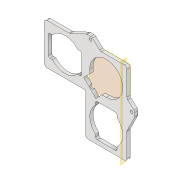
# Autodesk Inventor part: 20_Cube_Insert_Openflexure_Adapter
Saved by Autodesk Inventor 2019 (Build 230136000, 136)
## iProperties
Created: 2019-08-12
Part Number: 20_Cube_Insert_Openflexure_Adapter
Material: Generic
Document SubType Name: Modeling
Designer: diederichbenedict
Density: 1 g/cm^3
Appearance: White
Author: diederichbenedict
Autodesk Inventor part; units mm, degrees
ref_plane "YZ Plane" through (0, 0, 0) normal (1, 0, 0) x (0, 1, 0)
ref_plane "XZ Plane" through (0, 0, 0) normal (0, 1, 0) x (-1, 0, 0)
ref_plane "XY Plane" through (0, 0, 0) normal (0, 0, 1) x (1, 0, 0)
ref_plane "Work Plane1" through (0, 0, 0) normal (0, 0, 1) x (1, 0, 0)
sketch "Sketch1" plane through (0, 0, 0) normal (0, 0, 1) x (1, 0, 0)
  line L0 (-16.9, -16.9) -> (-16.9, 16.9) construction
  line L1 (-16.9, 16.9) -> (16.9, 16.9) construction
  line L2 (16.9, 16.9) -> (16.9, -16.9) construction
  line L3 (16.9, -16.9) -> (-16.9, -16.9) construction
  circle A0 centre (-19.9, 19.9) radius 2.75 construction
  circle A1 centre (19.9, -19.9) radius 2.75 construction
  circle A2 centre (19.9, 19.9) radius 2.75 construction
  circle A3 centre (-19.9, -19.9) radius 2.75 construction
  line L4 (-22.9, 22.9) -> (22.9, 22.9) construction
  line L5 (-22.9, -22.9) -> (-22.9, 22.9) construction
  line L6 (22.9, -22.9) -> (-22.9, -22.9) construction
  line L7 (22.9, 22.9) -> (22.9, -22.9) construction
  circle A4 centre (0, 0) radius 19.9847 construction
  circle A5 centre (30.6716, -19.9141) radius 1.6508 construction
  circle A6 centre (-19.2474, 31.0959) radius 1.649 construction
  line L8 (-11.1833, 28.6006) -> (11.7978, 28.3526) construction
  line L9 (-17.6359, 34.6452) -> (-11.1833, 28.6006) construction
  line L10 (-23.6485, 34.6452) -> (-17.6359, 34.6452) construction
  line L11 (-22.8713, 22.6559) -> (-23.6485, 34.6452) construction
  line L12 (-23.6485, -13.3567) -> (-22.8713, 22.6559) construction
  line L13 (-23.6485, -23.3548) -> (-23.6485, -13.3567) construction
  line L14 (34.3515, -23.3548) -> (-23.6485, -23.3548) construction
  line L15 (34.3515, -17.3548) -> (34.3515, -23.3548) construction
  line L16 (28.3526, -11.7978) -> (34.3515, -17.3548) construction
  line L17 (28.6006, 11.1833) -> (28.3526, -11.7978) construction
  arc A7 (28.6006, 11.1833) -> (11.7978, 28.3526) centre (10.7217, 10.4928) ccw construction
  arc A8 (-24.9, -22.9) -> (-22.9, -24.9) centre (-22.9, -22.9) ccw construction
  arc A9 (-22.9, 24.9) -> (-24.9, 22.9) centre (-22.9, 22.9) ccw construction
  arc A10 (24.9, 22.9) -> (22.9, 24.9) centre (22.9, 22.9) ccw construction
  arc A11 (22.9, -24.9) -> (24.9, -22.9) centre (22.9, -22.9) ccw construction
  line L18 (24.9, 24.9) -> (-74.9, 24.9) construction
  line L19 (-74.9, 24.9) -> (-74.9, -24.9) construction
  line L20 (-74.9, -24.9) -> (24.9, -24.9) construction
  line L21 (24.9, -24.9) -> (24.9, 24.9) construction
  line L22 (24.9, -24.9) -> (-25, -24.9) construction
  line L23 (-25, -24.9) -> (-25, -74.9) construction
  line L24 (-25, -74.9) -> (24.9, -74.9) construction
  line L25 (24.9, -74.9) -> (24.9, -24.9) construction
  line L26 (-74.9, 24.9) -> (-25, 24.9)
  line L27 (-25, 24.9) -> (-25, -24.9)
  line L28 (-25, -24.9) -> (-74.9, -24.9)
  line L29 (-74.9, -24.9) -> (-74.9, 24.9)
  line L30 (-25, -74.9) -> (24.9, -74.9)
  line L31 (24.9, -74.9) -> (24.9, -24.9)
  line L32 (24.9, -24.9) -> (-25, -24.9)
  line L33 (-25, -24.9) -> (-25, -74.9)
  circle A12 centre (0, 0) radius 20
  circle A13 centre (-50, 0) radius 20
  circle A14 centre (0, -50) radius 20
  line L34 (-25, -24.9) -> (24.9, -24.9)
  line L35 (24.9, -24.9) -> (24.9, 24.9)
  line L36 (24.9, 24.9) -> (-25, 24.9)
  line L37 (-25, 24.9) -> (-25, -24.9)
  line L38 (34.3515, -23.3548) -> (12.5761, -67.8407) construction
  line L39 (-24.6505, -24.1243) -> (34.3515, -23.3548) construction
  line L40 (-23.6485, 34.6452) -> (-24.6505, -24.1243) construction
  line L41 (-67.591, 14.0198) -> (-23.6485, 34.6452) construction
  arc A15 (-67.591, 14.0198) -> (-72.2252, 6.8961) centre (-64.1657, 6.7223) ccw construction
  line L42 (-72.3572, -5.3362) -> (-72.2252, 6.8961) construction
  arc A16 (-72.3572, -5.3362) -> (-70.7942, -10.6047) centre (-52.5572, -2.3284) ccw construction
  line L43 (-59.2435, -49.54) -> (-70.7942, -10.6047) construction
  line L44 (-50.8067, -58.1609) -> (-59.2435, -49.54) construction
  arc A17 (-50.8067, -58.1609) -> (-47.0776, -60.4156) centre (-44.5702, -52.0575) ccw construction
  line L45 (-6.8108, -72.2261) -> (-47.0776, -60.4156) construction
  arc A18 (-6.8108, -72.2261) -> (12.5761, -67.8407) centre (0.6863, -60.3238) ccw construction
  circle A19 centre (0, 0) radius 19.9847 construction
  circle A20 centre (-19.2474, 31.0959) radius 1.649 construction
  circle A21 centre (30.6716, -19.9141) radius 1.6508 construction
  line L46 (-11.1833, 28.6006) -> (11.7978, 28.3526) construction
  line L47 (-17.6359, 34.6452) -> (-11.1833, 28.6006) construction
  line L48 (-23.6485, 34.6452) -> (-17.6359, 34.6452) construction
  line L49 (-22.8713, 22.6559) -> (-23.6485, 34.6452) construction
  line L50 (-23.6485, -13.3567) -> (-22.8713, 22.6559) construction
  line L51 (-23.6485, -23.3548) -> (-23.6485, -13.3567) construction
  line L52 (34.3515, -23.3548) -> (-23.6485, -23.3548) construction
  line L53 (34.3515, -17.3548) -> (34.3515, -23.3548) construction
  line L54 (28.3526, -11.7978) -> (34.3515, -17.3548) construction
  line L55 (28.6006, 11.1833) -> (28.3526, -11.7978) construction
  arc A22 (28.6006, 11.1833) -> (11.7978, 28.3526) centre (10.7217, 10.4928) ccw construction
  line L56 (24.9, -42.6637) -> (34.3515, -23.3548)
  line L57 (34.3515, -23.3548) -> (34.3515, -17.3548)
  line L58 (34.3515, -17.3548) -> (24.9, -8.5995)
  line L59 (-17.6359, 34.6452) -> (-7.2331, 24.9)
  line L60 (-17.6359, 34.6452) -> (-23.6485, 34.6452)
  line L61 (-44.4107, 24.9) -> (-23.6485, 34.6452)
  circle A23 centre (-19.2474, 31.0959) radius 1.75
  circle A24 centre (30.6716, -19.9141) radius 1.75
  line L62 (-7.2331, 24.9) -> (-44.4107, 24.9)
  line L63 (-68, 13) -> (-32, 13)
  line L64 (-30, 11) -> (-30, -11)
  line L65 (-32, -13) -> (-68, -13)
  line L66 (-70, -11) -> (-70, 11)
  arc A25 (-68, 13) -> (-70, 11) centre (-68, 11) ccw
  arc A26 (-30, 11) -> (-32, 13) centre (-32, 11) ccw
  arc A27 (-32, -13) -> (-30, -11) centre (-32, -11) ccw
  arc A28 (-70, -11) -> (-68, -13) centre (-68, -11) ccw
  line L67 (24.9, 24.9) -> (-25, -25) construction
  line L68 (24.9, 24.9) -> (95.4693, 24.9) construction
  circle A29 centre (0, -50) radius 20
  arc A30 (6.8961, -72.2252) -> (14.0198, -67.591) centre (6.7223, -64.1657) ccw construction
  line L69 (-5.3362, -72.3572) -> (6.8961, -72.2252) construction
  arc A31 (-10.6047, -70.7942) -> (-5.3362, -72.3572) centre (-2.3284, -52.5572) ccw construction
  line L70 (13, -68) -> (13, -32)
  line L71 (11, -30) -> (-11, -30)
  line L72 (-13, -32) -> (-13, -68)
  line L73 (-11, -70) -> (11, -70)
  arc A32 (11, -70) -> (13, -68) centre (11, -68) ccw
  arc A33 (13, -32) -> (11, -30) centre (11, -32) ccw
  arc A34 (-11, -30) -> (-13, -32) centre (-11, -32) ccw
  arc A35 (-13, -68) -> (-11, -70) centre (-11, -68) ccw
  point P0 (0, 0)
  point P1 (-30, -13)
  point P2 (-30, 13)
  point P3 (-70, -13)
  point P4 (-13, -30)
  point P5 (13, -30)
  point P6 (-13, -70)
  dimension "d0" = 99.8
  dimension "d1" = 50
  dimension "d2" = 40
  dimension "d3" = 40
  dimension "d4" = 50
  dimension "d5" = 40
  dimension "d6" = 50
  dimension "d25" = 3.5
  dimension "d26" = 3.5
  dimension "d28" = 40
  dimension "d29" = 26
  dimension "d30" = 30
  dimension "d32" = 13
  dimension "d33" = 2
  dimension "d34" = 135
  constraints: 76 end point, 22 symmetric about line, 20 point on circle, 19 point on line, 16 centre point, 12 parallel, 8 tangent, 7 horizontal, 7 perpendicular, 3 coincident, 3 collinear, 3 equal radius, 1 equal length, 7 other
  measures "d0" distance of L20.end L19.end
  measures "d1" distance of L23.end L22.end
  measures "d2" diameter of A12
  measures "d3" diameter of A13
  measures "d4" distance of point (0, 0) A13.centre
  measures "d5" diameter of A14
  measures "d6" distance of A14.centre point (0, 0)
  measures "d25" diameter of A23
  measures "d26" diameter of A24
  measures "d28" distance of point (-30, -13) point (-70, -13)
  measures "d29" distance of point (-30, 13) point (-30, -13)
  measures "d30" distance from line of L64 A19.centre
  measures "d32" distance from line of L63 A19.centre
  measures "d33" radius of A25
  measures "d34" angle of L67 L68
extrude "Extrusion1" add sketch "Sketch1" along normal blind 4
ref_plane "Work Plane2" through (20, -74.9, 0) normal (1, 0, 0) x (0, 0, -1)
sketch "Sketch2" plane through (20, -74.9, 0) normal (1, 0, 0) x (0, 0, -1)
  line L0 (2.5, 97.55) -> (0, 97.55)
  line L1 (2.5, 92.05) -> (0, 92.05)
  line L2 (0, 94.9) -> (-4, 94.9) projected
  circle A0 centre (-1, 94.9) radius 2.45
  line L3 (1.45, 94.9) -> (-3.45, 94.9)
  line L4 (0, 0) -> (0, 99.8) construction
  point P0 (0, 74.9)
  dimension "d10" = 4.9
  dimension "d11" = 1
  constraints: 6 end point, 2 horizontal, 2 point on circle, 2 point on line, 1 centre point, 4 other
  measures "d10" diameter of A0
  measures "d11" distance from line of L4 A0.centre
revolve "Revolution1" cut sketch "Sketch2" angle 360 about axis through (20, 20, -1.45) along (0, 0, 1) picked at (-2.2763, 95.0954) contours L2 A0 L3
pattern_linear "Rectangular Pattern1" count 2 spacing 40 along (0, -1, 0) count 2 spacing 40 along (-1, 0, 0) of "Revolution1"
pattern_linear "Rectangular Pattern2" count 2 spacing 50 along (0, -1, 0) count 2 spacing 50 along (-1, 0, 0) of "Revolution1", "Rectangular Pattern1"
fillet "Fillet1" radius 3 14 edges at (-25, -24.9, 2) (-25, -74.9, 2) (24.9, -74.9, 2) (24.9, -42.6637, 2) (34.3515, -23.3548, 2) (34.3515, -17.3548, 2) (24.9, -8.5995, 2) (24.9, 24.9, 2) (-7.2331, 24.9, 2) (-17.6359, 34.6452, 2) (-23.6485, 34.6452, 2) (-44.4107, 24.9, 2) (-74.9, 24.9, 2) (-74.9, -24.9, 2)
sketch "Sketch3" plane through (0, 0, 4) normal (0, 0, 1) x (1, 0, 0)
  circle A0 centre (30.6716, -19.9141) radius 1.75 projected
  arc A1 (13, -65.1987) -> (13, -34.8013) centre (0, -50) ccw projected
  line L0 (13, -65.1987) -> (13, -68) projected
  arc A2 (11, -70) -> (13, -68) centre (11, -68) ccw projected
  line L1 (11, -70) -> (-11, -70) projected
  arc A3 (-13, -68) -> (-11, -70) centre (-11, -68) ccw projected
  line L2 (-13, -68) -> (-13, -65.1987) projected
  arc A4 (-13, -34.8013) -> (-13, -65.1987) centre (0, -50) ccw projected
  line L3 (-13, -34.8013) -> (-13, -32) projected
  arc A5 (-11, -30) -> (-13, -32) centre (-11, -32) ccw projected
  line L4 (-11, -30) -> (11, -30) projected
  arc A6 (13, -32) -> (11, -30) centre (11, -32) ccw projected
  line L5 (13, -32) -> (13, -34.8013) projected
  arc A7 (-65.1987, -13) -> (-34.8013, -13) centre (-50, 0) ccw projected
  line L6 (-65.1987, -13) -> (-68, -13) projected
  arc A8 (-70, -11) -> (-68, -13) centre (-68, -11) ccw projected
  line L7 (-70, -11) -> (-70, 11) projected
  arc A9 (-68, 13) -> (-70, 11) centre (-68, 11) ccw projected
  line L8 (-68, 13) -> (-65.1987, 13) projected
  arc A10 (-34.8013, 13) -> (-65.1987, 13) centre (-50, 0) ccw projected
  line L9 (-34.8013, 13) -> (-32, 13) projected
  arc A11 (-30, 11) -> (-32, 13) centre (-32, 11) ccw projected
  line L10 (-30, 11) -> (-30, -11) projected
  arc A12 (-32, -13) -> (-30, -11) centre (-32, -11) ccw projected
  line L11 (-32, -13) -> (-34.8013, -13) projected
  circle A13 centre (-19.2474, 31.0959) radius 1.75 projected
  circle A14 centre (0, 0) radius 20 projected
  arc A15 (-74.9, -21.9) -> (-71.9, -24.9) centre (-71.9, -21.9) ccw projected
  line L12 (-71.9, -24.9) -> (-28, -24.9) projected
  arc A16 (-25, -27.9) -> (-28, -24.9) centre (-28, -27.9) ccw projected
  line L13 (-25, -27.9) -> (-25, -71.9) projected
  arc A17 (-25, -71.9) -> (-22, -74.9) centre (-22, -71.9) ccw projected
  line L14 (-22, -74.9) -> (21.9, -74.9) projected
  arc A18 (21.9, -74.9) -> (24.9, -71.9) centre (21.9, -71.9) ccw projected
  line L15 (24.9, -71.9) -> (24.9, -43.3586) projected
  arc A19 (25.2055, -42.0396) -> (24.9, -43.3586) centre (27.9, -43.3586) ccw projected
  line L16 (25.2055, -42.0396) -> (34.046, -23.9789) projected
  arc A20 (34.046, -23.9789) -> (34.3515, -22.66) centre (31.3515, -22.66) ccw projected
  line L17 (34.3515, -22.66) -> (34.3515, -18.6652) projected
  arc A21 (34.3515, -18.6652) -> (33.3902, -16.4643) centre (31.3515, -18.6652) ccw projected
  line L18 (33.3902, -16.4643) -> (25.8613, -9.49) projected
  arc A22 (24.9, -7.2892) -> (25.8613, -9.49) centre (27.9, -7.2892) ccw projected
  line L19 (24.9, -7.2892) -> (24.9, 21.9) projected
  arc A23 (24.9, 21.9) -> (21.9, 24.9) centre (21.9, 21.9) ccw projected
  line L20 (21.9, 24.9) -> (-6.0474, 24.9) projected
  arc A24 (-8.0984, 25.7106) -> (-6.0474, 24.9) centre (-6.0474, 27.9) ccw projected
  line L21 (-8.0984, 25.7106) -> (-16.7706, 33.8346) projected
  arc A25 (-16.7706, 33.8346) -> (-18.8216, 34.6452) centre (-18.8216, 31.6452) ccw projected
  line L22 (-18.8216, 34.6452) -> (-22.9795, 34.6452) projected
  arc A26 (-22.9795, 34.6452) -> (-24.2541, 34.3609) centre (-22.9795, 31.6452) ccw projected
  line L23 (-24.2541, 34.3609) -> (-43.805, 25.1843) projected
  arc A27 (-45.0797, 24.9) -> (-43.805, 25.1843) centre (-45.0797, 27.9) ccw projected
  line L24 (-45.0797, 24.9) -> (-71.9, 24.9) projected
  arc A28 (-71.9, 24.9) -> (-74.9, 21.9) centre (-71.9, 21.9) ccw projected
  line L25 (-74.9, 21.9) -> (-74.9, -21.9) projected
  circle A29 centre (0, 0) radius 20 projected
  circle A30 centre (-20, -20) radius 2.2366 projected
  line L26 (-20, 0) -> (-20, -20)
  line L27 (-20, -20) -> (0, -20)
  line L28 (0, 0) -> (-20, 0)
  line L29 (-20, 0) -> (-20, -20)
  line L30 (-20, -20) -> (0, -20)
  line L31 (0, -20) -> (0, 0)
  line L32 (0, 0) -> (-14.1421, -14.1421)
  line L33 (0, 0) -> (20, 0) construction
  line L34 (13.2251, -1.5094) -> (-1.5094, 13.2251)
  line L35 (-1.5094, 13.2251) -> (-27.3673, -12.6327)
  line L36 (-27.3673, -12.6327) -> (-12.6327, -27.3673)
  line L37 (-12.6327, -27.3673) -> (13.2251, -1.5094)
  line L38 (13.2251, -1.5094) -> (-27.3673, -12.6327) construction
  line L39 (-1.5094, 13.2251) -> (-12.6327, -27.3673) construction
  point P0 (0, 0)
  point P1 (-7.0711, -7.0711)
  dimension "d37" = 135
  constraints: 28 end point, 4 midpoint, 4 parallel, 4 perpendicular, 2 horizontal, 2 point on circle, 1 equal length, 1 vertical, 1 vertical alignment, 1 other
  measures "d37" angle of L32 L33
extrude "Extrusion2" cut sketch "Sketch3" against normal blind 10 contours L28 L35 A14 | A14 L35 L26 | L27 L37 A14 | A14 L37 L31 | L35 L28 L32 A14 | A14 L37 L27 A30 L26 L35 | L26 A30 L36 L35 | L35 L34 L37 L31 L28 | A14 L32 L31 L37 | L37 L36 A30 L27 | L26 L36 A30 | A30 L27 L26 | A30 L36 L27
body "Solid1"
